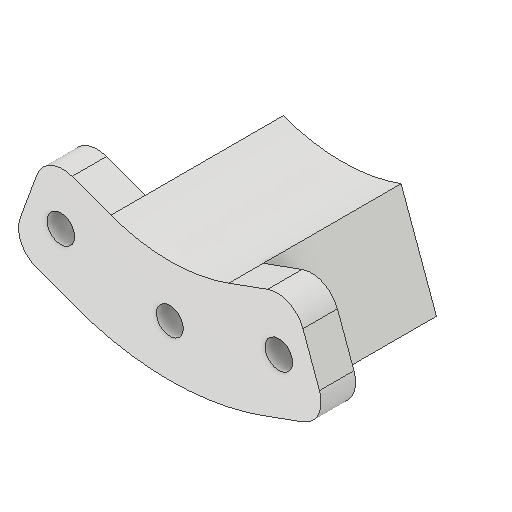
# Autodesk Inventor part: 3DP_ABS_Bowl_Feeder_Standoff
Saved by Autodesk Inventor 2026.1 (Build 301233000, 233)
## iProperties
Created: 2018-07-21
Part Number: 3DP_ABS_Bowl_Feeder_Standoff
Material: ABS Plastic
Document SubType Name: Modeling
Designer: Andrzej
Density: 1.06 g/cm^3
Appearance: Smooth - White
Author: Andrzej
Autodesk Inventor part; units mm, degrees
ref_plane "YZ Plane" through (0, 0, 0) normal (1, 0, 0) x (0, 1, 0)
ref_plane "XZ Plane" through (0, 0, 0) normal (0, 1, 0) x (-1, 0, 0)
ref_plane "XY Plane" through (0, 0, 0) normal (0, 0, 1) x (1, 0, 0)
sketch "Sketch1" plane through (0, 0, 0) normal (0, 0, 1) x (1, 0, 0)
  circle A0 centre (0, 0) radius 40
  circle A1 centre (0, 0) radius 32.5
  circle A2 centre (0, 0) radius 25
  line L0 (-8.5505, -23.4923) -> (-13.6808, -37.5877)
  line L1 (0, 0) -> (57.2098, 0) construction
  line L2 (8.5505, -23.4923) -> (13.6808, -37.5877)
  line L3 (0, 0) -> (61.497, 0) construction
  point P0 (0, -32.5)
  dimension "d1" = 65
  dimension "d0" = 80
  dimension "d2" = 50
  dimension "d4" = 110
  dimension "d6" = 70
  constraints: 8 end point, 4 point on circle, 3 coincident, 2 centre point, 2 horizontal, 1 vertical alignment, 2 other
  measures "d0" diameter of A0
  measures "d2" diameter of A2
  measures "d4" angle of L0 L1
  measures "d6" angle of L2 L3
extrude "Extrusion1" add sketch "Sketch1" along normal blind 20 contours L0 A1 L2 A0 | L0 A2 L2 A1 picked at (0, -34.8535) picked at (-0.9674, -29.7972)
sketch "Sketch2" plane through (0, 0, 20) normal (0, 0, 1) x (1, 0, 0)
  arc A0 (-13.6808, -37.5877) -> (13.6808, -37.5877) centre (0, 0) ccw projected
  line L0 (13.6808, -37.5877) -> (8.5505, -23.4923) projected
  arc A1 (-8.5505, -23.4923) -> (8.5505, -23.4923) centre (0, 0) ccw projected
  line L1 (-8.5505, -23.4923) -> (-13.6808, -37.5877) projected
  line L2 (8.5505, -23.4923) -> (17.9474, -20.0721)
  line L3 (17.9474, -20.0721) -> (23.0777, -34.1675)
  line L4 (23.0777, -34.1675) -> (13.6808, -37.5877)
  line L5 (-13.6808, -37.5877) -> (-23.0777, -34.1675)
  line L6 (-23.0777, -34.1675) -> (-17.9474, -20.0721)
  line L7 (-8.5505, -23.4923) -> (-13.6808, -37.5877) projected
  line L8 (-17.9474, -20.0721) -> (-8.5505, -23.4923)
  circle A2 centre (15.8141, -28.8299) radius 2
  circle A3 centre (-15.8141, -28.8299) radius 2
  dimension "d9" = 10
  dimension "d10" = 10
  dimension "d11" = 4
  dimension "d12" = 4
  dimension "d13" = 7.5
  dimension "d14" = 7.5
  dimension "d15" = 5
  dimension "d16" = 5
  constraints: 12 end point, 5 perpendicular, 2 centre point
  measures "d9" distance between parallel lines of L0 L3
  measures "d10" distance between parallel lines of L1 L6
  measures "d11" diameter of A2
  measures "d12" diameter of A3
  measures "d13" distance from line of L2 A2.centre
  measures "d14" distance from line of L8 A3.centre
  measures "d15" distance from line of L3 A2.centre
  measures "d16" distance from line of L6 A3.centre
extrude "Extrusion2" add sketch "Sketch2" along normal blind 5
chamfer "Chamfer1" distance 1.5 angle 45 2 edges at (-17.8141, -28.8299, 20) (13.8141, -28.8299, 20)
fillet "Fillet1" radius 4 4 edges at (17.9474, -20.0721, 22.5) (-17.9474, -20.0721, 22.5) (-23.0777, -34.1675, 22.5) (23.0777, -34.1675, 22.5)
hole "Hole1" at (0, -32.5, 0) direction (0, 0, 1) diameter 3.9 end through all
equation "\"d10\" = d9"
body "Solid1"
